Autodesk Fusion 360 part; units mm, degrees
note: some values were not read from the file. Set by a fixed rule: which sketch regions a step uses.
(part 4 of 4)
sketch "スケッチ32" plane through (0, 0, 3) normal (0, 0, 1) x (-1, 0, 0)
  arc A0 (-80.893, 31.3955) -> (-75.2362, 31.3955) centre (-78.0646, 34.224) ccw
  line L0 (-75.2362, 31.3955) -> (-66.5741, 40.0576)
  arc A1 (-63.7457, 40.0576) -> (-66.5741, 40.0576) centre (-65.1599, 38.6434) ccw
  line L1 (-63.7457, 40.0576) -> (-46.1401, 22.452)
  arc A2 (-45.7253, 20.2286) -> (-46.1401, 22.452) centre (-47.5543, 21.0378) ccw
  arc A3 (-45.7253, 20.2286) -> (-48.8685, 10.5769) centre (0, 0) ccw
  arc A4 (-50.8232, 9) -> (-48.8685, 10.5769) centre (-50.8232, 11) ccw
  line L2 (-50.8232, 9) -> (-96.3743, 9)
  arc A5 (-98.3614, 11.2268) -> (-96.3743, 9) centre (-96.3743, 11) ccw
  arc A6 (-91.4132, 38.0084) -> (-98.3614, 11.2268) centre (0, 0) ccw
  arc A7 (-88.1522, 38.6547) -> (-91.4132, 38.0084) centre (-89.5664, 37.2405) ccw
  line L3 (-88.1522, 38.6547) -> (-80.893, 31.3955)
  arc A8 (-31.3955, 75.2362) -> (-31.3955, 80.893) centre (-34.224, 78.0646) ccw
  line L4 (-31.3955, 80.893) -> (-38.6547, 88.1522)
  arc A9 (-38.0084, 91.4132) -> (-38.6547, 88.1522) centre (-37.2405, 89.5664) ccw
  arc A10 (-11.2268, 98.3614) -> (-38.0084, 91.4132) centre (0, 0) ccw
  arc A11 (-9, 96.3743) -> (-11.2268, 98.3614) centre (-11, 96.3743) ccw
  line L5 (-9, 96.3743) -> (-9, 50.8232)
  arc A12 (-10.5769, 48.8685) -> (-9, 50.8232) centre (-11, 50.8232) ccw
  arc A13 (-10.5769, 48.8685) -> (-20.2286, 45.7253) centre (0, 0) ccw
  arc A14 (-22.452, 46.1401) -> (-20.2286, 45.7253) centre (-21.0378, 47.5543) ccw
  line L6 (-22.452, 46.1401) -> (-40.0576, 63.7457)
  arc A15 (-40.0576, 66.5741) -> (-40.0576, 63.7457) centre (-38.6434, 65.1599) ccw
  line L7 (-40.0576, 66.5741) -> (-31.3955, 75.2362)
  arc A16 (31.3955, 80.893) -> (31.3955, 75.2362) centre (34.224, 78.0646) ccw
  line L8 (31.3955, 75.2362) -> (40.0576, 66.5741)
  arc A17 (40.0576, 63.7457) -> (40.0576, 66.5741) centre (38.6434, 65.1599) ccw
  line L9 (40.0576, 63.7457) -> (22.452, 46.1401)
  arc A18 (20.2286, 45.7253) -> (22.452, 46.1401) centre (21.0378, 47.5543) ccw
  arc A19 (20.2286, 45.7253) -> (10.5769, 48.8685) centre (0, 0) ccw
  arc A20 (9, 50.8232) -> (10.5769, 48.8685) centre (11, 50.8232) ccw
  line L10 (9, 50.8232) -> (9, 96.3743)
  arc A21 (11.2268, 98.3614) -> (9, 96.3743) centre (11, 96.3743) ccw
  arc A22 (38.0084, 91.4132) -> (11.2268, 98.3614) centre (0, 0) ccw
  arc A23 (38.6547, 88.1522) -> (38.0084, 91.4132) centre (37.2405, 89.5664) ccw
  line L11 (38.6547, 88.1522) -> (31.3955, 80.893)
  arc A24 (-5.7447, 44.6318) -> (-4, 46.6154) centre (-6, 46.6154) ccw
  line L12 (-4, 46.6154) -> (-4, 96.9794)
  arc A25 (-2.0412, 98.979) -> (-4, 96.9794) centre (-2, 96.9794) ccw
  arc A26 (2.0412, 98.979) -> (-2.0412, 98.979) centre (0, 0) ccw
  arc A27 (4, 96.9794) -> (2.0412, 98.979) centre (2, 96.9794) ccw
  line L13 (4, 96.9794) -> (4, 46.6154)
  arc A28 (4, 46.6154) -> (5.7447, 44.6318) centre (6, 46.6154) ccw
  arc A29 (28.3151, 34.9751) -> (5.7447, 44.6318) centre (0, 0) ccw
  arc A30 (28.4709, 32.0064) -> (28.3151, 34.9751) centre (27.0567, 33.4206) ccw
  line L14 (28.4709, 32.0064) -> (25.6252, 29.1607)
  arc A31 (22.9694, 29.007) -> (25.6252, 29.1607) centre (24.211, 30.575) ccw
  arc A32 (22.9694, 29.007) -> (-22.9694, 29.007) centre (0, 0) ccw
  arc A33 (-25.6252, 29.1607) -> (-22.9694, 29.007) centre (-24.211, 30.575) ccw
  line L15 (-25.6252, 29.1607) -> (-28.4709, 32.0064)
  arc A34 (-28.3151, 34.9751) -> (-28.4709, 32.0064) centre (-27.0567, 33.4206) ccw
  arc A35 (-5.7447, 44.6318) -> (-28.3151, 34.9751) centre (0, 0) ccw
  arc A36 (46.6154, -4) -> (44.6318, -5.7447) centre (46.6154, -6) ccw
  arc A37 (34.9751, -28.3151) -> (44.6318, -5.7447) centre (0, 0) ccw
  arc A38 (32.0064, -28.4709) -> (34.9751, -28.3151) centre (33.4206, -27.0567) ccw
  line L16 (32.0064, -28.4709) -> (29.1607, -25.6252)
  arc A39 (29.007, -22.9694) -> (29.1607, -25.6252) centre (30.575, -24.211) ccw
  arc A40 (29.007, -22.9694) -> (29.007, 22.9694) centre (0, 0) ccw
  arc A41 (29.1607, 25.6252) -> (29.007, 22.9694) centre (30.575, 24.211) ccw
  line L17 (29.1607, 25.6252) -> (32.0064, 28.4709)
  arc A42 (34.9751, 28.3151) -> (32.0064, 28.4709) centre (33.4206, 27.0567) ccw
  arc A43 (44.6318, 5.7447) -> (34.9751, 28.3151) centre (0, 0) ccw
  arc A44 (44.6318, 5.7447) -> (46.6154, 4) centre (46.6154, 6) ccw
  line L18 (46.6154, 4) -> (96.9794, 4)
  arc A45 (98.979, 2.0412) -> (96.9794, 4) centre (96.9794, 2) ccw
  arc A46 (98.979, -2.0412) -> (98.979, 2.0412) centre (0, 0) ccw
  arc A47 (96.9794, -4) -> (98.979, -2.0412) centre (96.9794, -2) ccw
  line L19 (96.9794, -4) -> (46.6154, -4)
  circle A48 centre (65.4951, -21.3591) radius 1.5
  circle A49 centre (57.7353, 37.5827) radius 1.5
  circle A50 centre (37.5827, 57.7353) radius 1.5
  circle A51 centre (-37.5827, 57.7353) radius 1.5
  circle A52 centre (-57.7353, 37.5827) radius 1.5
  circle A53 centre (-65.4951, -21.3591) radius 1.5
  circle A54 centre (51.2451, -46.0409) radius 1.5
  circle A55 centre (-51.2451, -46.0409) radius 1.5
  line L20 (-23, -28.9835) -> (-23, -22.2486)
  arc A56 (23.004, -22.2444) -> (-23, -22.2486) centre (0, 0) ccw
  line L21 (23.004, -22.2444) -> (23.004, -28.9802)
  arc A57 (25.6252, -29.1607) -> (23.004, -28.9802) centre (24.211, -30.575) ccw
  line L22 (25.6252, -29.1607) -> (28.4709, -32.0064)
  arc A58 (28.3151, -34.9751) -> (28.4709, -32.0064) centre (27.0567, -33.4206) ccw
  arc A59 (23.004, -38.6758) -> (28.3151, -34.9751) centre (0, 0) ccw
  line L23 (23.004, -38.6758) -> (23.004, -40.172)
  line L24 (23.004, -40.172) -> (27.273, -42.6405)
  arc A60 (28.1158, -41.3462) -> (27.273, -42.6405) centre (29.2404, -43) ccw
  arc A61 (28.1158, -41.3462) -> (31.3739, -38.9317) centre (0, 0) ccw
  arc A62 (33.6289, -38.7569) -> (31.3739, -38.9317) centre (32.6289, -40.4889) ccw
  line L25 (33.6289, -38.7569) -> (37.9782, -41.268)
  arc A63 (36.9782, -45) -> (37.9782, -41.268) centre (36.9782, -43) ccw
  line L26 (36.9782, -45) -> (31.3533, -45)
  line L27 (31.3533, -45) -> (40, -50)
  line L28 (40, -50) -> (38, -50)
  arc A64 (40, -52) -> (38, -50) centre (38, -52) ccw
  line L29 (40, -52) -> (40, -56)
  arc A65 (38, -58) -> (40, -56) centre (38, -56) ccw
  line L30 (38, -58) -> (-38, -58)
  arc A66 (-40, -56) -> (-38, -58) centre (-38, -56) ccw
  line L31 (-40, -56) -> (-40, -52)
  arc A67 (-38, -50) -> (-40, -52) centre (-38, -52) ccw
  line L32 (-38, -50) -> (-40, -50)
  line L33 (-40, -50) -> (-31.3513, -45)
  line L34 (-31.3513, -45) -> (-36.9782, -45)
  arc A68 (-37.9782, -41.2679) -> (-36.9782, -45) centre (-36.9782, -43) ccw
  line L35 (-37.9782, -41.2679) -> (-33.6289, -38.7569)
  arc A69 (-31.3739, -38.9317) -> (-33.6289, -38.7569) centre (-32.6289, -40.4889) ccw
  arc A70 (-31.3739, -38.9317) -> (-28.1158, -41.3462) centre (0, 0) ccw
  arc A71 (-27.2727, -42.6421) -> (-28.1158, -41.3462) centre (-29.2404, -43) ccw
  line L36 (-27.2727, -42.6421) -> (-23, -40.172)
  line L37 (-23, -40.172) -> (-23, -38.6782)
  arc A72 (-28.3589, -34.9396) -> (-23, -38.6782) centre (0, 0) ccw
  arc A73 (-28.4908, -31.9509) -> (-28.3589, -34.9396) centre (-27.0985, -33.3867) ccw
  line L38 (-28.4908, -31.9509) -> (-25.5966, -29.1445)
  arc A74 (-23, -28.9835) -> (-25.5966, -29.1445) centre (-24.2043, -30.5803) ccw
  line L39 (-78.4041, -8.9935) -> (-56.6098, -9.0353)
  arc A75 (-55.6136, -12.7673) -> (-56.6098, -9.0353) centre (-56.6136, -11.0353) ccw
  line L40 (-55.6136, -12.7673) -> (-71.9413, -22.1941)
  arc A76 (-74.6733, -21.462) -> (-71.9413, -22.1941) centre (-72.9413, -20.462) ccw
  line L41 (-74.6733, -21.462) -> (-80.14, -11.9935)
  arc A77 (-78.4041, -8.9935) -> (-80.14, -11.9935) centre (-78.4079, -10.9935) ccw
  line L42 (50.1096, -15.3631) -> (69.4413, -26.5242)
  arc A78 (70.1733, -29.2563) -> (69.4413, -26.5242) centre (68.4413, -28.2563) ccw
  line L43 (70.1733, -29.2563) -> (60.4233, -46.1437)
  arc A79 (57.6913, -46.8758) -> (60.4233, -46.1437) centre (58.6913, -45.1437) ccw
  line L44 (57.6913, -46.8758) -> (38.3596, -35.7147)
  arc A80 (37.8458, -32.6756) -> (38.3596, -35.7147) centre (39.3596, -33.9826) ccw
  arc A81 (37.8458, -32.6756) -> (47.2208, -16.4376) centre (0, 0) ccw
  arc A82 (50.1096, -15.3631) -> (47.2208, -16.4376) centre (49.1096, -17.0951) ccw
  line L45 (-44.4259, 27.8089) -> (-60.2101, 43.5931)
  arc A83 (-60.2101, 46.4216) -> (-60.2101, 43.5931) centre (-58.7959, 45.0073) ccw
  line L46 (-60.2101, 46.4216) -> (-46.4216, 60.2101)
  arc A84 (-43.5931, 60.2101) -> (-46.4216, 60.2101) centre (-45.0073, 58.7959) ccw
  line L47 (-43.5931, 60.2101) -> (-27.8089, 44.4259)
  arc A85 (-28.0992, 41.3574) -> (-27.8089, 44.4259) centre (-29.2231, 43.0117) ccw
  arc A86 (-28.0992, 41.3574) -> (-41.3574, 28.0992) centre (0, 0) ccw
  arc A87 (-44.4259, 27.8089) -> (-41.3574, 28.0992) centre (-43.0117, 29.2231) ccw
  line L48 (80.1362, -12) -> (74.6733, -21.462)
  arc A88 (71.9413, -22.1941) -> (74.6733, -21.462) centre (72.9413, -20.462) ccw
  line L49 (71.9413, -22.1941) -> (55.6136, -12.7673)
  arc A89 (56.6098, -9.0353) -> (55.6136, -12.7673) centre (56.6136, -11.0353) ccw
  line L50 (56.6098, -9.0353) -> (75, -9)
  line L51 (75, -9) -> (78.4042, -9)
  arc A90 (80.1362, -12) -> (78.4042, -9) centre (78.4042, -11) ccw
  line L52 (-38.3596, -35.7147) -> (-57.6913, -46.8758)
  arc A91 (-60.4233, -46.1437) -> (-57.6913, -46.8758) centre (-58.6913, -45.1437) ccw
  line L53 (-60.4233, -46.1437) -> (-70.1733, -29.2563)
  arc A92 (-69.4413, -26.5242) -> (-70.1733, -29.2563) centre (-68.4413, -28.2563) ccw
  line L54 (-69.4413, -26.5242) -> (-50.1096, -15.3631)
  arc A93 (-47.2208, -16.4376) -> (-50.1096, -15.3631) centre (-49.1096, -17.0951) ccw
  arc A94 (-47.2208, -16.4376) -> (-37.8458, -32.6756) centre (0, 0) ccw
  arc A95 (-38.3596, -35.7147) -> (-37.8458, -32.6756) centre (-39.3596, -33.9826) ccw
  line L55 (27.8089, 44.4259) -> (43.5931, 60.2101)
  arc A96 (46.4216, 60.2101) -> (43.5931, 60.2101) centre (45.0073, 58.7959) ccw
  line L56 (46.4216, 60.2101) -> (60.2101, 46.4216)
  arc A97 (60.2101, 43.5931) -> (60.2101, 46.4216) centre (58.7959, 45.0073) ccw
  line L57 (60.2101, 43.5931) -> (44.4259, 27.8089)
  arc A98 (41.3574, 28.0992) -> (44.4259, 27.8089) centre (43.0117, 29.2231) ccw
  arc A99 (41.3574, 28.0992) -> (28.0992, 41.3574) centre (0, 0) ccw
  arc A100 (27.8089, 44.4259) -> (28.0992, 41.3574) centre (29.2231, 43.0117) ccw
  arc A101 (-44.6318, -5.7447) -> (-46.6154, -4) centre (-46.6154, -6) ccw
  line L58 (-46.6154, -4) -> (-96.9794, -4)
  arc A102 (-98.979, -2.0412) -> (-96.9794, -4) centre (-96.9794, -2) ccw
  arc A103 (-98.979, 2.0412) -> (-98.979, -2.0412) centre (0, 0) ccw
  arc A104 (-96.9794, 4) -> (-98.979, 2.0412) centre (-96.9794, 2) ccw
  line L59 (-96.9794, 4) -> (-46.6154, 4)
  arc A105 (-46.6154, 4) -> (-44.6318, 5.7447) centre (-46.6154, 6) ccw
  arc A106 (-34.9648, 28.3278) -> (-44.6318, 5.7447) centre (0, 0) ccw
  arc A107 (-31.975, 28.4611) -> (-34.9648, 28.3278) centre (-33.4108, 27.0688) ccw
  line L60 (-31.975, 28.4611) -> (-29.1682, 25.5666)
  arc A108 (-29.0345, 22.9346) -> (-29.1682, 25.5666) centre (-30.604, 24.1743) ccw
  arc A109 (-29.0345, 22.9346) -> (-29.007, -22.9694) centre (0, 0) ccw
  arc A110 (-29.1607, -25.6252) -> (-29.007, -22.9694) centre (-30.575, -24.211) ccw
  line L61 (-29.1607, -25.6252) -> (-32.0064, -28.4709)
  arc A111 (-34.9751, -28.3151) -> (-32.0064, -28.4709) centre (-33.4206, -27.0567) ccw
  arc A112 (-44.6318, -5.7447) -> (-34.9751, -28.3151) centre (0, 0) ccw
  line L62 (-96.3722, -9.0182) -> (-93.084, -9.0182)
  arc A113 (-92.084, -12.7502) -> (-93.084, -9.0182) centre (-93.084, -11.0182) ccw
  line L63 (-92.084, -12.7502) -> (-95.1531, -14.5221)
  arc A114 (-98.1356, -13.0538) -> (-95.1531, -14.5221) centre (-96.1531, -12.7901) ccw
  arc A115 (-98.3593, -11.2453) -> (-98.1356, -13.0538) centre (0, 0) ccw
  arc A116 (-96.3722, -9.0182) -> (-98.3593, -11.2453) centre (-96.3722, -11.0182) ccw
  arc A117 (98.1356, -13.0538) -> (98.3593, -11.2453) centre (0, 0) ccw
  arc A118 (95.1531, -14.5221) -> (98.1356, -13.0538) centre (96.1531, -12.7901) ccw
  line L64 (95.1531, -14.5221) -> (92.084, -12.7502)
  arc A119 (93.084, -9.0182) -> (92.084, -12.7502) centre (93.084, -11.0182) ccw
  line L65 (93.084, -9.0182) -> (96.3722, -9.0182)
  arc A120 (98.3593, -11.2453) -> (96.3722, -9.0182) centre (96.3722, -11.0182) ccw
  arc A121 (76.6504, 29.9813) -> (79.4788, 29.9813) centre (78.0646, 31.3955) ccw
  line L66 (79.4788, 29.9813) -> (88.1522, 38.6547)
  arc A122 (91.4132, 38.0084) -> (88.1522, 38.6547) centre (89.5664, 37.2405) ccw
  arc A123 (98.3614, 11.2268) -> (91.4132, 38.0084) centre (0, 0) ccw
  arc A124 (96.3743, 9) -> (98.3614, 11.2268) centre (96.3743, 11) ccw
  line L67 (96.3743, 9) -> (50.8232, 9)
  arc A125 (48.8685, 10.5769) -> (50.8232, 9) centre (50.8232, 11) ccw
  arc A126 (48.8685, 10.5769) -> (45.7253, 20.2286) centre (0, 0) ccw
  arc A127 (46.1401, 22.452) -> (45.7253, 20.2286) centre (47.5543, 21.0378) ccw
  line L68 (46.1401, 22.452) -> (63.7457, 40.0576)
  arc A128 (66.5741, 40.0576) -> (63.7457, 40.0576) centre (65.1599, 38.6434) ccw
  line L69 (66.5741, 40.0576) -> (76.6504, 29.9813)
  line L70 (-52.5666, -50) -> (-47, -50)
  arc A129 (-45, -52) -> (-47, -50) centre (-47, -52) ccw
  line L71 (-45, -52) -> (-45, -62)
  arc A130 (-47, -64) -> (-45, -62) centre (-47, -62) ccw
  line L72 (-47, -64) -> (-48.9593, -64)
  arc A131 (-50.6914, -63) -> (-48.9593, -64) centre (-48.9593, -62) ccw
  line L73 (-50.6914, -63) -> (-55.9233, -53.938)
  arc A132 (-55.1913, -51.2059) -> (-55.9233, -53.938) centre (-54.1913, -52.938) ccw
  line L74 (-55.1913, -51.2059) -> (-53.5666, -50.2679)
  arc A133 (-52.5666, -50) -> (-53.5666, -50.2679) centre (-52.5666, -52) ccw
  line L75 (55.9233, -53.938) -> (50.6914, -63)
  arc A134 (48.9593, -64) -> (50.6914, -63) centre (48.9593, -62) ccw
  line L76 (48.9593, -64) -> (47, -64)
  arc A135 (45, -62) -> (47, -64) centre (47, -62) ccw
  line L77 (45, -62) -> (45, -51.9629)
  arc A136 (46.9625, -49.9632) -> (45, -51.9629) centre (47, -51.9629) ccw
  line L78 (46.9625, -49.9632) -> (52.2919, -49.8634)
  arc A137 (53.3294, -50.131) -> (52.2919, -49.8634) centre (52.3294, -51.863) ccw
  line L79 (53.3294, -50.131) -> (55.1913, -51.2059)
  arc A138 (55.9233, -53.938) -> (55.1913, -51.2059) centre (54.1913, -52.938) ccw
  arc A139 (54.7686, -84) -> (67.0189, -79.5265) centre (54.7686, -64.99) ccw
  arc A140 (67.0189, -79.5265) -> (67.021, -79.5248) centre (0, 0) ccw
  arc A141 (67.021, -79.5248) -> (66.4432, -73.002) centre (64.4432, -76.4661) ccw
  line L80 (66.4432, -73.002) -> (56.3605, -67.1808)
  arc A142 (55.6284, -64.4487) -> (56.3605, -67.1808) centre (57.3605, -65.4487) ccw
  line L81 (55.6284, -64.4487) -> (83.6284, -15.9513)
  arc A143 (86.3605, -15.2192) -> (83.6284, -15.9513) centre (85.3605, -16.9513) ccw
  line L82 (86.3605, -15.2192) -> (96.4432, -21.0405)
  arc A144 (96.4432, -21.0405) -> (102.381, -18.2795) centre (98.4432, -17.5764) ccw
  arc A145 (102.381, -18.2795) -> (94.1613, 44.1547) centre (0, 0) ccw
  arc A146 (94.1613, 44.1547) -> (87.7113, 45.2849) centre (90.5398, 42.4565) ccw
  line L83 (87.7113, 45.2849) -> (79.4788, 37.0524)
  arc A147 (76.6504, 37.0524) -> (79.4788, 37.0524) centre (78.0646, 38.4666) ccw
  line L84 (76.6504, 37.0524) -> (37.0524, 76.6504)
  arc A148 (37.0524, 79.4788) -> (37.0524, 76.6504) centre (38.4666, 78.0646) ccw
  line L85 (37.0524, 79.4788) -> (45.2849, 87.7113)
  arc A149 (45.2849, 87.7113) -> (44.1547, 94.1613) centre (42.4565, 90.5398) ccw
  arc A150 (44.1547, 94.1613) -> (-44.1547, 94.1613) centre (0, 0) ccw
  arc A151 (-44.1547, 94.1613) -> (-45.2849, 87.7113) centre (-42.4565, 90.5398) ccw
  line L86 (-45.2849, 87.7113) -> (-37.0524, 79.4788)
  arc A152 (-37.0524, 76.6504) -> (-37.0524, 79.4788) centre (-38.4666, 78.0646) ccw
  line L87 (-37.0524, 76.6504) -> (-76.6504, 37.0524)
  arc A153 (-79.4788, 37.0524) -> (-76.6504, 37.0524) centre (-78.0646, 38.4666) ccw
  line L88 (-79.4788, 37.0524) -> (-87.7113, 45.2849)
  arc A154 (-87.7113, 45.2849) -> (-94.1613, 44.1547) centre (-90.5398, 42.4565) ccw
  arc A155 (-94.1613, 44.1547) -> (-102.381, -18.2795) centre (0, 0) ccw
  arc A156 (-102.381, -18.2795) -> (-96.4432, -21.0405) centre (-98.4432, -17.5764) ccw
  line L89 (-96.4432, -21.0405) -> (-86.3605, -15.2192)
  arc A157 (-83.6284, -15.9513) -> (-86.3605, -15.2192) centre (-85.3605, -16.9513) ccw
  line L90 (-83.6284, -15.9513) -> (-55.6284, -64.4487)
  arc A158 (-56.3605, -67.1808) -> (-55.6284, -64.4487) centre (-57.3605, -65.4487) ccw
  line L91 (-56.3605, -67.1808) -> (-66.4432, -73.002)
  arc A159 (-66.4432, -73.002) -> (-67.021, -79.5248) centre (-64.4432, -76.4661) ccw
  arc A160 (-67.021, -79.5248) -> (-67.0189, -79.5265) centre (0.0001, 0.0001) ccw
  arc A161 (-67.0189, -79.5265) -> (-54.7686, -84) centre (-54.7686, -64.99) ccw
  line L92 (-54.7686, -84) -> (-44, -84)
  arc A162 (-44, -84) -> (-40, -80) centre (-44, -80) ccw
  line L93 (-40, -80) -> (-40, -66)
  arc A163 (-38, -64) -> (-40, -66) centre (-38, -66) ccw
  line L94 (-38, -64) -> (38, -64)
  arc A164 (40, -66) -> (38, -64) centre (38, -66) ccw
  line L95 (40, -66) -> (40, -80)
  arc A165 (40, -80) -> (44, -84) centre (44, -80) ccw
  line L96 (44, -84) -> (54.7686, -84)
  line L97 (35.8035, -40.0124) -> (34.8035, -41.7445)
  line L98 (34.8035, -41.7445) -> (22.8227, -34.8273)
  line L99 (34.8035, -41.7445) -> (48.9736, -49.9256)
  line L100 (40, -50) -> (48.9736, -49.9256)
  line L101 (-35.8035, -40.0124) -> (-34.8035, -41.7445)
  line L102 (-34.8035, -41.7445) -> (-22.4341, -34.603)
  line L103 (-34.8035, -41.7445) -> (-49.1025, -50)
  line L104 (-49.1025, -50) -> (-40, -50)
  line L105 (-40, -50) -> (-23, -40.172)
  line L106 (-23, -40.172) -> (-23, -34.9297)
  line L107 (40, -50) -> (23.004, -40.172)
  line L108 (23.004, -40.172) -> (23.004, -34.932)
  dimension "d206" = 2
  dimension "d207" = 2
  constraint midpoint L25 L97.start
  constraint perpendicular L25 L97
  constraint perpendicular L97 L98
  constraint coincident L78 L99.end
  constraint perpendicular L97 L99
  constraint coincident L27.end L28.start
  constraint midpoint L35 L101.start
  constraint perpendicular L35 L101
  constraint perpendicular L101 L102
  constraint coincident L70 L103.end
  constraint perpendicular L101 L103
  constraint coincident L32.end L33.start
  constraint coincident L36.end L37.start
  constraint coincident L102 L106.end
  constraint parallel L37 L106
  constraint coincident L23.end L24.start
  constraint coincident L98 L108.end
  constraint parallel L23 L108
  measures "d206" distance of L97.start L97.end
  measures "d207" distance of L101.start L101.end
extrude "押し出し31" add sketch "スケッチ32" along normal blind 1.6 contours A72 L102 L106 | A70 A71 L36 L37 A72 L102 L105 L106 | L34 A68 A70 A71 L102 L103 L105 | A59 L23 L24 A60 A61 L98 L107 L108 | A59 L98 L108 | L33 L34 A68 L70 L103 L104 L105 | A60 A61 A63 L26 L98 L99 L107 | A63 L26 L27 L99 L100 L107 bodies 1
extrude "押し出し32" cut 1 faces at (51.5716, 78.2876, 1.5) along direction (0, 0, 1) blind 1.5 on bodies 1 bodies 1
fillet "フィレット34" radius 2 6 edges at (-48.9736, 49.9256, 3.8) (49.1025, 50, 3.8) (-23.004, 34.932, 3.8) (-23.004, -16, 3.8) (23, -16, 3.8) (23, 34.9297, 3.8) on bodies 1
sketch "スケッチ33" plane through (0, 0, 4.6) normal (0, 0, 1) x (-1, 0, 0)
  arc A0 (-21, 16) -> (-23, 14) centre (-21, 14) ccw
  line L0 (-23, 14) -> (-23, -33.775)
  arc A1 (-24, -35.507) -> (-23, -33.775) centre (-25, -33.775) ccw
  line L1 (-24, -35.507) -> (-42.6384, -46.2679)
  arc A2 (-42.6384, -46.2679) -> (-41.6384, -50) centre (-41.6384, -48) ccw
  line L2 (-41.6384, -50) -> (-40, -50)
  line L3 (-40, -50) -> (40, -50)
  line L4 (40, -50) -> (41.6317, -49.9865)
  arc A3 (41.6317, -49.9865) -> (42.6151, -46.2545) centre (41.6151, -47.9865) ccw
  line L5 (42.6151, -46.2545) -> (24.004, -35.5094)
  arc A4 (23.004, -33.7773) -> (24.004, -35.5094) centre (25.004, -33.7773) ccw
  line L6 (23.004, -33.7773) -> (23.004, 14)
  arc A5 (23.004, 14) -> (21.004, 16) centre (21.004, 14) ccw
  line L7 (21.004, 16) -> (0.004, 16)
  line L8 (0.004, 16) -> (-21, 16)
  circle A6 centre (0, 0) radius 32
  constraint coincident A6.centre origin
extrude "押し出し33" add sketch "スケッチ33" against normal blind 1.6 contours A0 L0 L6 A5 L7 L8 A6 picked at (-11.7036, 20.2396) bodies 1
sketch "スケッチ34" plane through (0, 0, 4.6) normal (0, 0, 1) x (-1, 0, 0)
  line L0 (-23, -22.2486) -> (-23, -33.775)
  arc A0 (-24, -35.507) -> (-23, -33.775) centre (-25, -33.775) ccw
  line L1 (-24, -35.507) -> (-42.6384, -46.2679)
  arc A1 (-42.6384, -46.2679) -> (-41.6384, -50) centre (-41.6384, -48) ccw
  line L2 (-41.6384, -50) -> (-40, -50)
  line L3 (-40, -50) -> (40, -50)
  line L4 (40, -50) -> (41.6317, -49.9865)
  arc A2 (41.6317, -49.9865) -> (42.6151, -46.2545) centre (41.6151, -47.9865) ccw
  line L5 (42.6151, -46.2545) -> (24.004, -35.5094)
  arc A3 (23.004, -33.7773) -> (24.004, -35.5094) centre (25.004, -33.7773) ccw
  line L6 (23.004, -33.7773) -> (23.004, -22.2444)
  arc A4 (23.004, -22.2444) -> (-23, -22.2486) centre (0, 0) ccw
  line L7 (-41.6384, -48) -> (-43.6384, -48)
  line L8 (-43.6384, -48) -> (-43.6384, -43)
  line L9 (41.6151, -47.9865) -> (43.6151, -47.9865)
  line L10 (43.6151, -47.9865) -> (43.6151, -42.9865)
  line L11 (-43.6384, -43) -> (-23, -31.0844)
  line L12 (43.6151, -42.9865) -> (23.004, -31.0844)
  dimension "d216" = 5
  dimension "d217" = 5
  constraint coincident A1.centre L7.start
  constraint coincident A1 L7.end
  constraint horizontal L7
  constraint perpendicular L7 L8
  constraint coincident A2.centre L9.start
  constraint coincident A2 L9.end
  constraint horizontal L9
  constraint perpendicular L9 L10
  constraint coincident L0 L11.end
  constraint parallel L1 L11
  constraint coincident L6 L12.end
  measures "d216" distance of L7.end L8.end
  measures "d217" distance of L9.end L10.end
extrude "押し出し34" add sketch "スケッチ34" against normal blind 1.6 contours L0 A0 L1 A1 L8 L11 | A2 L5 A3 L6 L10 L12 bodies 1
fillet "フィレット35" radius 2 2 edges at (23, 31.0844, 3.8) (23, 22.2486, 3.8) on bodies 1
fillet "フィレット36" radius 2 1 edges at (43.6384, 43, 3.8) on bodies 1
fillet "フィレット37" radius 2 3 edges at (-43.6151, 42.9865, 3.8) (-23.004, 22.2444, 3.8) (-23.004, 31.0844, 3.8) on bodies 1
sketch "スケッチ35" plane through (0, 0, 4.6) normal (0, 0, 1) x (-1, 0, 0)
  arc A0 (43.6151, -44.1411) -> (42.6153, -42.4092) centre (41.6151, -44.1411) ccw
  line L0 (42.6153, -42.4092) -> (24.0039, -31.6618)
  arc A1 (23.004, -29.9298) -> (24.0039, -31.6618) centre (25.004, -29.9298) ccw
  line L1 (23.004, -29.9298) -> (23.004, -23.039)
  arc A2 (23.5332, -21.6838) -> (23.004, -23.039) centre (25.004, -23.039) ccw
  arc A3 (23.5332, -21.6838) -> (-23.5294, -21.6879) centre (0, 0) ccw
  arc A4 (-23, -23.0434) -> (-23.5294, -21.6879) centre (-25, -23.0434) ccw
  line L2 (-23, -23.0434) -> (-23, -29.9297)
  arc A5 (-24, -31.6617) -> (-23, -29.9297) centre (-25, -29.9297) ccw
  line L3 (-24, -31.6617) -> (-42.6384, -42.4226)
  arc A6 (-42.6384, -42.4226) -> (-43.6384, -44.1547) centre (-41.6384, -44.1547) ccw
  line L4 (-43.6384, -44.1547) -> (-43.6384, -48)
  arc A7 (-43.6384, -48) -> (-41.6384, -50) centre (-41.6384, -48) ccw
  line L5 (-41.6384, -50) -> (-40, -50)
  line L6 (-40, -50) -> (40, -50)
  line L7 (40, -50) -> (41.6317, -49.9865)
  arc A8 (41.6317, -49.9865) -> (43.6151, -47.9865) centre (41.6151, -47.9865) ccw
  line L8 (43.6151, -47.9865) -> (43.6151, -44.1411)
  line L9 (0, 0) -> (0, 16)
  line L10 (0, 16) -> (-14, 16)
  line L11 (0, 16) -> (14, 16)
  line L12 (14, 16) -> (14, 28.775)
  line L13 (-14, 16) -> (-14, 28.775)
  dimension "d226" = 16
  dimension "d227" = 14
  dimension "d228" = 14
  constraint coincident A3.centre L9.start
  constraint vertical L9
  constraint perpendicular L9 L10
  constraint perpendicular L9 L11
  constraint coincident A3 L12.end
  constraint perpendicular L11 L12
  constraint coincident A3 L13.end
  constraint perpendicular L11 L13
  measures "d226" distance of A3.centre L9.end
  measures "d227" distance of L9.end L10.end
  measures "d228" distance of L9.end L11.end
extrude "押し出し35" cut sketch "スケッチ35" against normal blind 10 contours A3 L10 L11 L12 L13 bodies 1
fillet "フィレット38" radius 2 4 edges at (-14, -16, 3.8) (-14, -28.775, 3.8) (14, -28.775, 3.8) (14, -16, 3.8) on bodies 1
